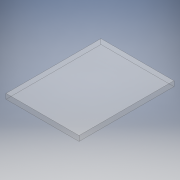
# Autodesk Inventor part: Frente inferior - porta1
Saved by Autodesk Inventor 2017 (Build 210142000, 142)
## iProperties
Created: 2016-08-19
Part Number: Frente inferior - porta1
Material: Polycarbonate, Clear
Document SubType Name: Modeling
Designer: Alunos
Density: 1.2 g/cm^3
Appearance: Polycarbonate - Clear
Author: Alunos
Autodesk Inventor part; units mm, degrees
ref_plane "YZ Plane" through (0, 0, 0) normal (1, 0, 0) x (0, 1, 0)
ref_plane "XZ Plane" through (0, 0, 0) normal (0, 1, 0) x (-1, 0, 0)
ref_plane "XY Plane" through (0, 0, 0) normal (0, 0, 1) x (1, 0, 0)
sketch "Sketch1" plane through (0, 0, 0) normal (0, 0, 1) x (1, 0, 0)
  line L0 (0, 0) -> (100, 0)
  line L1 (100, 0) -> (100, 130)
  line L2 (100, 130) -> (0, 130)
  line L3 (0, 130) -> (0, 0)
  dimension "d0" = 100
  dimension "d1" = 130
  constraints: 8 end point, 2 parallel, 1 horizontal, 1 perpendicular
  measures "d0" distance of L2.end L1.end
  measures "d1" distance of L1.end L0.end
extrude "Extrusion1" add sketch "Sketch1" along normal blind 7
body "Solid1"
